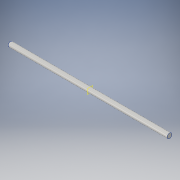
# Autodesk Inventor part: dualLiftAxel
Saved by Autodesk Inventor 2016 SP1 (Build 200210100, 210)
## iProperties
Created: 2016-02-03
Part Number: dualLiftAxel
Material: Aluminum 6061
Document SubType Name: Modeling
Designer: steele
Mass: 145.516 g
Surface Area: 172.281 cm^2
Volume: 53.8947 cm^3
Density: 2.7 g/cm^3
Appearance: Aluminum - Flat
Author: steele
Autodesk Inventor part; units mm, degrees
ref_plane "XZ Plane" through (0, 0, 0) normal (0, 1, 0) x (-1, 0, 0)
ref_plane "XY Plane" through (0, 0, 0) normal (0, 0, 1) x (1, 0, 0)
sketch "Sketch1" plane through (0, 0, 0) normal (1, 0, 0) x (0, 1, 0)
  circle A0 centre (0, 0) radius 6.35
  dimension "d0" = 12.7
  constraints: 1 centre point, 1 coincident
  measures "d0" diameter of A0
extrude "Extrusion1" add sketch "Sketch1" along normal mid plane 425.45
equation "\"d0\" = axelDiam"
equation "\"d1\" = axelLength"
equation "\"axelDiam\" = 12.7"
equation "\"axelLength\" = 425.45"
body "Solid1"
